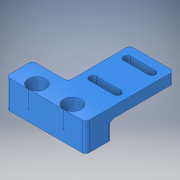
# Autodesk Inventor part: Belt_Clamp_R
Saved by Autodesk Inventor 2019.4 (Build 234330000, 330)
## iProperties
Created: 2021-02-15
Part Number: Belt_Clamp_R
Material: ABS Plastic
Document SubType Name: Modeling
Designer: Jorian Brusind
Density: 1.06 g/cm^3
Appearance: Cyan
Author: Jorian Brusind
Autodesk Inventor part; units mm, degrees
ref_plane "YZ Plane" through (0, 0, 0) normal (1, 0, 0) x (0, 1, 0)
ref_plane "XZ Plane" through (0, 0, 0) normal (0, 1, 0) x (-1, 0, 0)
ref_plane "XY Plane" through (0, 0, 0) normal (0, 0, 1) x (1, 0, 0)
sketch "Sketch1" plane through (0, 0, 0) normal (0, 1, 0) x (-1, 0, 0)
  line L0 (0, 0) -> (-45, 0)
  line L1 (-45, 0) -> (-45, -50)
  line L2 (-45, -50) -> (0, -50)
  line L3 (0, -50) -> (0, 0)
  line L4 (0, -50) -> (-20, -50)
  line L5 (-20, -50) -> (-20, -15)
  line L6 (-20, -15) -> (0, -15)
  line L7 (0, -15) -> (0, -50)
  dimension "d0" = 45
  dimension "d1" = 50
  dimension "d2" = 20
  dimension "d3" = 35
  constraints: 16 end point, 4 parallel, 2 horizontal, 2 perpendicular
  measures "d0" distance of L2.end L1.end
  measures "d1" distance of L1.end L0.end
  measures "d2" distance of L5.end L6.end
  measures "d3" distance of L4.end L5.end
extrude "Extrusion1" add sketch "Sketch1" along normal blind 6 contours L3 L6 L5 L2 L1 L0
sketch "Sketch2" plane through (0, 6, 0) normal (0, 1, 0) x (1, 0, 0)
  line L0 (25.5, 43) -> (39.5, 43) construction
  line L1 (25.5, 41) -> (39.5, 41)
  line L2 (39.5, 45) -> (25.5, 45)
  arc A0 (25.5, 45) -> (25.5, 41) centre (25.5, 43) ccw
  arc A1 (39.5, 41) -> (39.5, 45) centre (39.5, 43) ccw
  line L3 (32.5, 43) -> (46.5, 43) construction
  line L4 (45, 0) -> (45, 50) projected
  line L5 (45, 50) -> (20, 50) projected
  line L6 (25.5, 23.5) -> (39.5, 23.5) construction
  line L7 (25.5, 21.5) -> (39.5, 21.5)
  line L8 (39.5, 25.5) -> (25.5, 25.5)
  arc A2 (25.5, 25.5) -> (25.5, 21.5) centre (25.5, 23.5) ccw
  arc A3 (39.5, 21.5) -> (39.5, 25.5) centre (39.5, 23.5) ccw
  line L9 (32.5, 23.5) -> (46.5, 23.5) construction
  point P0 (0, 0)
  dimension "d6" = 7
  dimension "d7" = 0
  dimension "d8" = 4
  dimension "d9" = 5.5
  dimension "d10" = 5
  dimension "d11" = 7
  dimension "d12" = 0
  dimension "d13" = 4
  dimension "d14" = 5.5
  dimension "d15" = 19.5
  constraints: 20 end point, 8 point on circle, 8 tangent, 4 centre point, 4 horizontal, 2 collinear, 2 midpoint, 2 parallel
  measures "d6" distance of L3.start L0.end
  measures "d7" distance between parallel lines of L0 L3
  measures "d8" diameter of A1
  measures "d9" distance from line of L4 L0.end
  measures "d10" distance between parallel lines of L5 L2
  measures "d11" distance of L9.start L6.end
  measures "d12" distance between parallel lines of L6 L9
  measures "d13" diameter of A3
  measures "d14" distance from line of L4 L6.end
  measures "d15" distance between parallel lines of L0 L6
extrude "Extrusion2" cut sketch "Sketch2" against normal up to next
sketch "Sketch4" plane through (0, 0, 0) normal (0, -1, 0) x (1, 0, 0)
  line L0 (0, -15) -> (0, 0) projected
  line L1 (0, 0) -> (45, 0)
  line L2 (45, 0) -> (45, -15)
  line L3 (45, -15) -> (0, -15)
  line L4 (0, -15) -> (0, 0)
  dimension "d18" = 45
  dimension "d19" = 15
  constraints: 8 end point, 2 parallel, 1 horizontal, 1 perpendicular
  measures "d18" distance of L2.end L3.end
  measures "d19" distance of L1.end L2.end
extrude "Extrusion3" add sketch "Sketch4" along normal blind 10
sketch "Sketch3" plane through (0, 6, 0) normal (0, 1, 0) x (1, 0, 0)
  circle A0 centre (12.5, 5) radius 2.75
  circle A1 centre (32.5, 5) radius 2.75
  line L0 (45, 0) -> (45, 50) projected
  line L1 (0, 0) -> (45, 0) projected
  dimension "d22" = 5.5
  dimension "d23" = 5.5
  dimension "d24" = 12.5
  dimension "d25" = 5
  dimension "d26" = 5
  dimension "d27" = 20
  constraints: 2 centre point
  measures "d22" diameter of A0
  measures "d23" diameter of A1
  measures "d24" distance from line of L0 A1.centre
  measures "d25" distance from line of L1 A1.centre
  measures "d26" distance from line of L1 A0.centre
  measures "d27" distance of A1.centre A0.centre
extrude "Extrusion4" cut sketch "Sketch3" against normal up to next
sketch "Sketch5" plane through (0, 6, 0) normal (0, 1, 0) x (1, 0, 0)
  circle A0 centre (12.5, 5) radius 2.75 projected
  circle A1 centre (12.5, 5) radius 5
  circle A2 centre (32.5, 5) radius 2.75 projected
  circle A3 centre (32.5, 5) radius 5
  point P0 (0, 0)
  dimension "d30" = 10
  dimension "d31" = 10
  constraints: 2 centre point, 2 coincident
  measures "d30" diameter of A1
  measures "d31" diameter of A3
extrude "Extrusion5" cut sketch "Sketch5" against normal blind 10
fillet "Fillet1" radius 2 8 edges at (0, -2, 0) (45, -2, 0) (0, -2, -15) (20, 3, -15) (32.5, 0, -15) (45, 3, -50) (20, 3, -50) (45, -5, -15)
body "Solid1"
